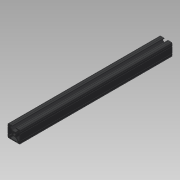
# Autodesk Inventor part: 1001-BLACK-FB
Saved by Autodesk Inventor 2013 (Build 170138000, 138)
## iProperties
Company: 80/20 Inc.
Created: 2014-04-23
Part Number: 1001-BLACK-FB
Material: Generic
Document SubType Name: Modeling
Density: 1 g/cm^3
Vendor: 80/20 Inc.
Engineer: Ross Bowman
Designer: Ross Bowman
Catalog Web Link: 8020.net
Material: 6105-T5 Aluminum
Author: Ross Bowman
Keywords: 80/20 , 8020 , T-Slot , Extrusion
Autodesk Inventor part; units mm, degrees
ref_plane "YZ Plane" through (0, 0, 0) normal (1, 0, 0) x (0, 1, 0)
ref_plane "XZ Plane" through (0, 0, 0) normal (0, 1, 0) x (-1, 0, 0)
ref_plane "XY Plane" through (0, 0, 0) normal (0, 0, 1) x (1, 0, 0)
sketch "Sketch1" plane through (0, 0, 0) normal (0, 0, 1) x (1, 0, 0)
  arc A0 (-1.6262, -4.5044) -> (-3.8713, -5.4343) centre (-1.6262, -7.6794) ccw
  line L0 (1.6262, -4.5044) -> (-1.6262, -4.5044)
  arc A1 (3.8713, -5.4343) -> (1.6262, -4.5044) centre (1.6262, -7.6794) ccw
  line L1 (7.1551, -8.7181) -> (3.8713, -5.4343)
  arc A2 (6.3985, -10.4902) -> (7.1551, -8.7181) centre (6.3689, -9.43) ccw
  line L2 (-6.4049, -10.4902) -> (6.3985, -10.4902)
  arc A3 (-7.1552, -8.7184) -> (-6.4049, -10.4902) centre (-6.369, -9.4302) ccw
  line L3 (-3.8713, -5.4343) -> (-7.1552, -8.7184)
  circle A4 centre (0, 0) radius 2.6035
  arc A5 (-4.5044, 1.6262) -> (-5.4343, 3.8713) centre (-7.6794, 1.6262) ccw
  line L4 (-4.5044, -1.6262) -> (-4.5044, 1.6262)
  arc A6 (-5.4343, -3.8713) -> (-4.5044, -1.6262) centre (-7.6794, -1.6262) ccw
  line L5 (-8.7181, -7.1551) -> (-5.4343, -3.8713)
  arc A7 (-10.4902, -6.3985) -> (-8.7181, -7.1551) centre (-9.43, -6.3689) ccw
  line L6 (-10.4902, 6.4049) -> (-10.4902, -6.3985)
  arc A8 (-8.7184, 7.1552) -> (-10.4902, 6.4049) centre (-9.4302, 6.369) ccw
  line L7 (-5.4343, 3.8713) -> (-8.7184, 7.1552)
  arc A9 (8.7184, -7.1552) -> (10.4902, -6.4049) centre (9.4302, -6.369) ccw
  line L8 (5.4343, -3.8713) -> (8.7184, -7.1552)
  arc A10 (4.5044, -1.6262) -> (5.4343, -3.8713) centre (7.6794, -1.6262) ccw
  line L9 (4.5044, 1.6262) -> (4.5044, -1.6262)
  arc A11 (5.4343, 3.8713) -> (4.5044, 1.6262) centre (7.6794, 1.6262) ccw
  line L10 (8.7181, 7.1551) -> (5.4343, 3.8713)
  arc A12 (10.4902, 6.3985) -> (8.7181, 7.1551) centre (9.43, 6.3689) ccw
  line L11 (10.4902, -6.4049) -> (10.4902, 6.3985)
  arc A13 (12.7, -9.5504) -> (12.7, -10.5664) centre (12.7, -10.0584) ccw
  line L12 (12.7, -9.5504) -> (12.7, -6.604)
  arc A14 (12.7, -5.588) -> (12.7, -6.604) centre (12.7, -6.096) ccw
  line L13 (12.7, -5.588) -> (12.7, 5.588)
  arc A15 (12.7, 6.604) -> (12.7, 5.588) centre (12.7, 6.096) ccw
  line L14 (12.7, 6.604) -> (12.7, 9.5504)
  arc A16 (12.7, 10.5664) -> (12.7, 9.5504) centre (12.7, 10.0584) ccw
  line L15 (12.7, 10.5664) -> (12.7, 10.5918)
  arc A17 (12.7, 10.5918) -> (10.5918, 12.7) centre (10.5918, 10.5918) ccw
  line L16 (10.5918, 12.7) -> (10.5664, 12.7)
  arc A18 (9.5504, 12.7) -> (10.5664, 12.7) centre (10.0584, 12.7) ccw
  line L17 (9.5504, 12.7) -> (6.604, 12.7)
  arc A19 (5.588, 12.7) -> (6.604, 12.7) centre (6.096, 12.7) ccw
  line L18 (5.588, 12.7) -> (4.3561, 12.7)
  arc A20 (4.3561, 12.7) -> (4.3561, 10.4902) centre (4.3561, 11.5951) ccw
  line L19 (4.3561, 10.4902) -> (6.4049, 10.4902)
  arc A21 (7.1552, 8.7184) -> (6.4049, 10.4902) centre (6.369, 9.4302) ccw
  line L20 (7.1552, 8.7184) -> (3.8713, 5.4343)
  arc A22 (1.6262, 4.5044) -> (3.8713, 5.4343) centre (1.6262, 7.6794) ccw
  line L21 (1.6262, 4.5044) -> (-1.6262, 4.5044)
  arc A23 (-3.8713, 5.4343) -> (-1.6262, 4.5044) centre (-1.6262, 7.6794) ccw
  line L22 (-3.8713, 5.4343) -> (-7.1551, 8.7181)
  arc A24 (-6.3985, 10.4902) -> (-7.1551, 8.7181) centre (-6.3689, 9.43) ccw
  line L23 (-6.3985, 10.4902) -> (-4.3561, 10.4902)
  arc A25 (-4.3561, 10.4902) -> (-4.3561, 12.7) centre (-4.3561, 11.5951) ccw
  line L24 (-4.3561, 12.7) -> (-5.588, 12.7)
  arc A26 (-6.604, 12.7) -> (-5.588, 12.7) centre (-6.096, 12.7) ccw
  line L25 (-6.604, 12.7) -> (-9.5504, 12.7)
  arc A27 (-10.5664, 12.7) -> (-9.5504, 12.7) centre (-10.0584, 12.7) ccw
  line L26 (-10.5664, 12.7) -> (-10.5918, 12.7)
  arc A28 (-10.5918, 12.7) -> (-12.7, 10.5918) centre (-10.5918, 10.5918) ccw
  line L27 (-12.7, 10.5918) -> (-12.7, 10.5664)
  arc A29 (-12.7, 9.5504) -> (-12.7, 10.5664) centre (-12.7, 10.0584) ccw
  line L28 (-12.7, 9.5504) -> (-12.7, 6.604)
  arc A30 (-12.7, 5.588) -> (-12.7, 6.604) centre (-12.7, 6.096) ccw
  line L29 (-12.7, 5.588) -> (-12.7, -5.588)
  arc A31 (-12.7, -6.604) -> (-12.7, -5.588) centre (-12.7, -6.096) ccw
  line L30 (-12.7, -6.604) -> (-12.7, -9.5504)
  arc A32 (-12.7, -10.5664) -> (-12.7, -9.5504) centre (-12.7, -10.0584) ccw
  line L31 (-12.7, -10.5664) -> (-12.7, -10.5918)
  arc A33 (-12.7, -10.5918) -> (-10.5918, -12.7) centre (-10.5918, -10.5918) ccw
  line L32 (-10.5918, -12.7) -> (-10.5664, -12.7)
  arc A34 (-9.5504, -12.7) -> (-10.5664, -12.7) centre (-10.0584, -12.7) ccw
  line L33 (-9.5504, -12.7) -> (-6.604, -12.7)
  arc A35 (-5.588, -12.7) -> (-6.604, -12.7) centre (-6.096, -12.7) ccw
  line L34 (-5.588, -12.7) -> (5.588, -12.7)
  arc A36 (6.604, -12.7) -> (5.588, -12.7) centre (6.096, -12.7) ccw
  line L35 (6.604, -12.7) -> (9.5504, -12.7)
  arc A37 (10.5664, -12.7) -> (9.5504, -12.7) centre (10.0584, -12.7) ccw
  line L36 (10.5664, -12.7) -> (10.5918, -12.7)
  arc A38 (10.5918, -12.7) -> (12.7, -10.5918) centre (10.5918, -10.5918) ccw
  line L37 (12.7, -10.5918) -> (12.7, -10.5664)
  constraints: 76 end point, 76 point on circle, 39 centre point
extrude "Extrusion1" add sketch "Sketch1" against normal blind 304.8
body "Solid1"
